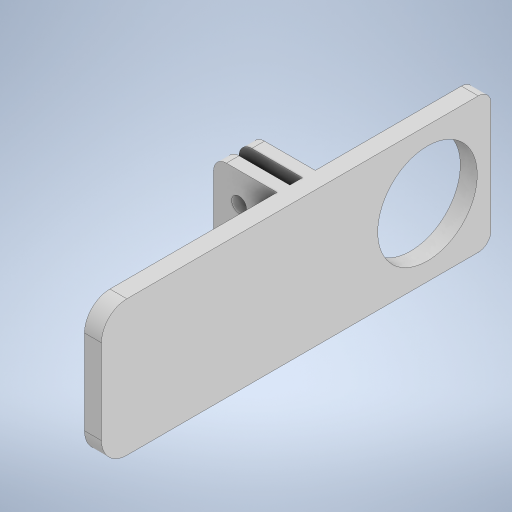
# Autodesk Inventor part: POUPLY_P5_V2
Saved by Autodesk Inventor 2024 (Build 280153000, 153)
## iProperties
Created: 2024-04-22
Part Number: POUPLY_P5_V2
Material: Generic
Document SubType Name: Modeling
Designer: luc4s
Density: 1 g/cm^3
Appearance: Default
Author: luc4s
Autodesk Inventor part; units mm, degrees
ref_plane "YZ Plane" through (0, 0, 0) normal (1, 0, 0) x (0, 1, 0)
ref_plane "XZ Plane" through (0, 0, 0) normal (0, 1, 0) x (-1, 0, 0)
ref_plane "XY Plane" through (0, 0, 0) normal (0, 0, 1) x (1, 0, 0)
sketch "Sketch1" plane through (0, 0, 0) normal (1, 0, 0) x (0, 1, 0)
  line L0 (16, 50) -> (-16, 50)
  line L1 (-16, 50) -> (-16, -42)
  line L2 (-16, -42) -> (16, -42)
  line L3 (16, -42) -> (16, 50)
  circle A0 centre (0, -27) radius 11.75
  line L4 (0, 0) -> (0, -82.2599) construction
  dimension "d0" = 23.5
  dimension "d1" = 27
  dimension "d2" = 50
  dimension "d3" = 32
  dimension "d5" = 42
  constraints: 10 end point, 2 parallel, 1 centre point, 1 horizontal, 1 perpendicular, 1 point on line, 1 vertical, 1 other
  measures "d0" diameter of A0
  measures "d1" distance of L4.start A0.centre
  measures "d2" distance from line of L4.start L0
  measures "d3" distance of L1.end L2.end
  measures "d5" vertical distance of L4.start L1.end
extrude "Extrusion1" add sketch "Sketch1" along normal blind 4
fillet "Fillet1" radius 3 2 edges at (2, -16, -42) (2, 16, -42)
fillet "Fillet2" radius 6 1 edges at (2, -16, 50)
fillet "Fillet3" radius 6 1 edges at (2, 16, 50)
sketch "Sketch2" plane through (0, 0, 0) normal (-1, 0, 0) x (0, 0, 1)
  line L0 (44, -16) -> (-39, -16) projected
  line L1 (-39, 16) -> (44, 16) projected
  line L2 (-1.5, -16) -> (-4.5, -16)
  line L3 (-4.5, -16) -> (-4.5, 16)
  line L4 (-4.5, 16) -> (-1.5, 16)
  line L5 (-1.5, 16) -> (-1.5, -16)
  line L6 (1.5, 16) -> (4.5, 16)
  line L7 (4.5, 16) -> (4.5, -16)
  line L8 (4.5, -16) -> (1.5, -16)
  line L9 (1.5, -16) -> (1.5, 16)
  line L10 (0, -16) -> (0, 16) construction
  point P0 (0, 0)
  point P1 (-1.5, 16)
  point P2 (1.5, 16)
  point P3 (1.5, -16)
  point P4 (4.5, -16)
  dimension "d11" = 3
  dimension "d12" = 3
  dimension "d13" = 3
  constraints: 18 end point, 6 point on line, 4 parallel, 3 perpendicular, 2 horizontal, 1 midpoint, 1 other
  measures "d11" distance between parallel lines of L9 L7
  measures "d12" distance between parallel lines of L3 L5
  measures "d13" distance between parallel lines of L5 L9
extrude "Extrusion2" add sketch "Sketch2" along normal blind 15 contours L0 L9 L1 L7 | L0 L3 L1 L5
fillet "Fillet4" radius 3 4 edges at (-15, -16, 3) (-15, -16, -3) (-15, 16, 3) (-15, 16, -3)
sketch "Sketch3" plane through (0, -16, -4.5) normal (0, 0, -1) x (-1, 0, 0)
  circle A0 centre (9, 7) radius 1.75
  circle A1 centre (9, 25) radius 1.75
  line L0 (0, 0) -> (12, 0) projected
  line L1 (0, 32) -> (12, 32) projected
  line L2 (15, 29) -> (15, 3) projected
  circle A2 centre (5, 16) radius 1.75
  point P0 (0, 16)
  dimension "d17" = 3.5
  dimension "d18" = 3.5
  dimension "d19" = 7
  dimension "d20" = 7
  dimension "d21" = 6
  dimension "d22" = 6
  dimension "d23" = 16
  dimension "d24" = 10
  dimension "d25" = 3.5
  constraints: 3 centre point
  measures "d17" diameter of A0
  measures "d18" diameter of A1
  measures "d19" distance from line of L0 A0.centre
  measures "d20" distance from line of L1 A1.centre
  measures "d21" distance from line of L2 A1.centre
  measures "d22" distance from line of L2 A0.centre
  measures "d23" distance from line of L0 A2.centre
  measures "d24" distance from line of L2 A2.centre
  measures "d25" diameter of A2
extrude "Extrusion3" cut sketch "Sketch3" against normal blind 15
body "Solid1"
